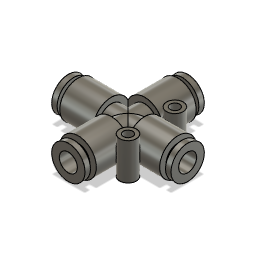
Top+Hydraulics (Autodesk Fusion 360 archive; units mm, degrees)
design "Cross Tube Fitting"
Autodesk Fusion 360 part; units mm, degrees
sketch "Sketch1" plane through (0, 0, 0) normal (0, 1, 0) x (1, 0, 0)
  line L0 (0, 21) -> (0, 0)
  line L1 (0, 21) -> (-5.875, 21)
  line L2 (-5.875, 21) -> (-5.875, 19.08)
  line L3 (-5.875, 19.08) -> (-4.175, 19.08)
  line L4 (-4.175, 19.08) -> (-4.175, 17.58)
  line L5 (-4.175, 17.58) -> (-6.45, 17.58)
  line L6 (-6.45, 17.58) -> (-6.45, 5.88)
  line L7 (-6.45, 5.88) -> (-4.475, 5.88)
  line L8 (-4.475, 5.88) -> (-4.475, 0)
  line L9 (-4.475, 0) -> (0, 0)
  line L10 (2.5, 0) -> (20, 0)
  line L11 (-5.875, -21) -> (-5.875, -19.08)
  line L12 (-6.45, -17.58) -> (-6.45, -5.88)
  line L13 (-4.175, -19.08) -> (-4.175, -17.58)
  line L14 (-5.875, -19.08) -> (-4.175, -19.08)
  line L15 (-6.45, -5.88) -> (-4.475, -5.88)
  line L16 (0, -21) -> (-5.875, -21)
  line L17 (-4.175, -17.58) -> (-6.45, -17.58)
  line L18 (0, -21) -> (0, 0)
  line L19 (-4.475, -5.88) -> (-4.475, 0)
  dimension "d1" = 21
  dimension "d2" = 5.875
  dimension "d3" = 1.92
  dimension "d4" = 1.7
  dimension "d5" = 1.5
  dimension "d6" = 2.275
  dimension "d7" = 11.7
  dimension "d8" = 5.88
  dimension "d9" = 4.475
  constraint coincident L0.end L9.end
  constraint perpendicular L0 L1
  constraint perpendicular L1 L2
  constraint perpendicular L2 L3
  constraint perpendicular L3 L4
  constraint perpendicular L4 L5
  constraint perpendicular L5 L6
  constraint perpendicular L6 L7
  constraint perpendicular L0 L9
  constraint parallel L9 L10
  constraint symmetric L0.start L9 L16.start
  constraint symmetric L0.end L9 L18.end
  constraint symmetric L1.end L9 L11.start
  constraint symmetric L2.end L9 L11.end
  constraint symmetric L3.end L9 L13.start
  constraint symmetric L4.end L9 L13.end
  constraint symmetric L5.end L9 L12.start
  constraint symmetric L6.end L9 L12.end
  constraint symmetric L7.end L9 L15.end
  constraint symmetric L8.end L9 L19.end
  measures "d1" distance of L0.start L0.end
  measures "d2" distance of L0.start L1.end
  measures "d3" distance of L1.end L2.end
  measures "d4" distance of L2.end L3.end
  measures "d5" distance of L3.end L4.end
  measures "d6" distance of L4.end L5.end
  measures "d7" distance of L5.end L6.end
  measures "d8" distance of L7.end L8.end
  measures "d9" distance of L0.end L8.end
revolve "Revolve1" add sketch "Sketch1" angle 360 about axis through (0, 0, 21) along (0, 0, -1)
sketch "Sketch2" plane through (0, 0, 0) normal (0, 1, 0) x (1, 0, 0)
  line L0 (19.08, 4.175) -> (17.58, 4.175)
  line L1 (5.88, 4.475) -> (0, 4.475)
  line L2 (21, 0) -> (21, 5.875)
  line L3 (21, 5.875) -> (19.08, 5.875)
  line L4 (5.88, 6.45) -> (5.88, 4.475)
  line L5 (0, 4.475) -> (0, 0)
  line L6 (17.58, 6.45) -> (5.88, 6.45)
  line L7 (21, 0) -> (0, 0)
  line L8 (17.58, 4.175) -> (17.58, 6.45)
  line L9 (19.08, 5.875) -> (19.08, 4.175)
  line L10 (0, 21) -> (0, 0)
  line L11 (-21, 0) -> (0, 0)
  line L12 (-17.58, 4.175) -> (-17.58, 6.45)
  line L13 (-5.88, 6.45) -> (-5.88, 4.475)
  line L14 (-19.08, 5.875) -> (-19.08, 4.175)
  line L15 (-17.58, 6.45) -> (-5.88, 6.45)
  line L16 (0, 4.475) -> (0, 0)
  line L17 (-19.08, 4.175) -> (-17.58, 4.175)
  line L18 (-21, 0) -> (-21, 5.875)
  line L19 (-21, 5.875) -> (-19.08, 5.875)
  line L20 (-5.88, 4.475) -> (0, 4.475)
  line L21 (2.5, 0) -> (20, 0)
  line L22 (0, -20) -> (0, -2.5)
  point P0 (0, 4.475)
  point P1 (0, 4.475)
  dimension "d11" = 21
  dimension "d12" = 5.875
  dimension "d13" = 1.92
  dimension "d14" = 1.7
  dimension "d15" = 1.5
  dimension "d16" = 2.275
  dimension "d17" = 11.7
  dimension "d18" = 5.88
  dimension "d19" = 4.475
  constraint coincident L5.end L7.end
  constraint perpendicular L2 L7
  constraint perpendicular L2 L3
  constraint perpendicular L3 L9
  constraint perpendicular L0 L9
  constraint perpendicular L0 L8
  constraint perpendicular L6 L8
  constraint perpendicular L4 L6
  constraint perpendicular L5 L7
  constraint symmetric L7.end L10.end L5
  constraint symmetric P1 P0 L5
  constraint symmetric L5.end L10 L7.end
  constraint symmetric L1.start L10 L13.end
  constraint symmetric L4.start L10 L13.start
  constraint symmetric L0.end L10 L12.start
  constraint symmetric L2.start L10 L11.start
  constraint symmetric L0.start L10 L14.end
  constraint symmetric L2.end L10 L18.end
  constraint symmetric L3.end L10 L14.start
  constraint symmetric P1 L10 P0
  constraint symmetric L6.start L10 L12.end
  constraint parallel L7 L11
  measures "d11" distance of L2.start L5.end
  measures "d12" distance of L2.start L2.end
  measures "d13" distance of L2.end L3.end
  measures "d14" distance of L0.start L3.end
  measures "d15" distance of L0.end L0.start
  measures "d16" distance of L0.end L6.start
  measures "d17" distance of L4.start L6.start
  measures "d18" distance of L1.start P0
  measures "d19" distance of P1 L5.end
revolve "Revolve2" add sketch "Sketch2" angle 360 about axis through (21, 0, 0) along (-1, 0, 0)
sketch "Sketch3" plane through (21, 0, 0) normal (1, 0, 0) x (0, 0, -1)
  circle A0 centre (0, 0) radius 5.875
  circle A1 centre (0, 0) radius 3.175
  dimension "d21" = 6.35
  constraint coincident A0.centre A1.centre
  measures "d21" diameter of A1
extrude "Extrude1" cut sketch "Sketch3" against normal up to surface (42 mm away) contours A1
sketch "Sketch4" plane through (0, 0, -21) normal (0, 0, -1) x (-1, 0, 0)
  circle A0 centre (0, 0) radius 5.875
  circle A1 centre (0, 0) radius 3.175
  dimension "d24" = 6.35
  constraint coincident A0.centre A1.centre
  measures "d24" diameter of A1
extrude "Extrude2" cut sketch "Sketch4" against normal up to surface (42 mm away) contours A1
sketch "Sketch5" plane through (0, 0, 0) normal (0, 1, 0) x (1, 0, 0)
  line L0 (0, -20) -> (0, -2.5)
  circle A0 centre (8.25, -8.25) radius 1.65
  line L1 (2.5, 0) -> (20, 0)
  circle A1 centre (8.25, -8.25) radius 2.95
  circle A2 centre (8.25, 8.25) radius 1.65
  circle A3 centre (8.25, 8.25) radius 2.95
  dimension "d27" = 3.3
  dimension "d28" = 8.25
  dimension "d29" = 8.25
  dimension "d30" = 5.9
  constraint concentric A0 A1
  constraint symmetric A0 L1 A2
  constraint symmetric L1 A1 A3
  measures "d27" diameter of A0
  measures "d28" distance of L0 A0.centre
  measures "d29" distance of A0.centre L1
  measures "d30" diameter of A1
extrude "Extrude3" add sketch "Sketch5" along normal mid plane 12.9

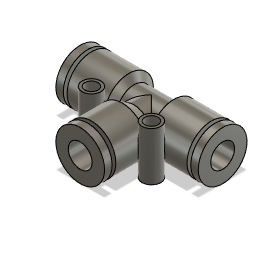
design "Marine 3-Way Push-to-Connect"
Autodesk Fusion 360 part; units mm, degrees
sketch "Sketch1" plane through (0, 0, 0) normal (0, 1, 0) x (1, 0, 0)
  line L0 (0, -20) -> (0, -2.5)
  line L1 (0, 3.18) -> (19, 3.18)
  line L2 (2.5, 0) -> (20, 0)
  line L3 (19, 3.18) -> (19, 6.5)
  line L4 (0, 4.55) -> (4.65, 4.55)
  line L5 (4.65, 4.55) -> (6, 6.5)
  line L6 (17, 6.5) -> (17, 3.75)
  line L7 (17, 3.75) -> (16, 3.75)
  line L8 (16, 3.75) -> (16, 6.5)
  line L9 (19, 6.5) -> (17, 6.5)
  line L10 (16, 6.5) -> (6, 6.5)
  line L11 (0, 4.55) -> (-4.65, 4.55)
  line L12 (0, 3.18) -> (-19, 3.18)
  line L13 (-4.65, 4.55) -> (-6, 6.5)
  line L14 (-16, 6.5) -> (-6, 6.5)
  line L15 (-16, 3.75) -> (-16, 6.5)
  line L16 (-17, 6.5) -> (-17, 3.75)
  line L17 (-17, 3.75) -> (-16, 3.75)
  line L18 (-19, 6.5) -> (-17, 6.5)
  line L19 (-19, 3.18) -> (-19, 6.5)
  dimension "d2" = 19
  dimension "d3" = 3.18
  dimension "d4" = 6.5
  dimension "d5" = 6
  dimension "d6" = 4.65
  dimension "d7" = 4.55
  dimension "d8" = 1
  dimension "d9" = 2
  dimension "d10" = 2.75
  constraint horizontal L1
  constraint coincident L0 L1.start
  constraint perpendicular L1 L3
  constraint perpendicular L3 L9
  constraint horizontal L4
  constraint perpendicular L6 L9
  constraint perpendicular L3 L7
  constraint coincident L8.end L9
  constraint perpendicular L8 L9
  constraint collinear L9 L10
  constraint symmetric L0 L1.start L12.start
  constraint symmetric L0 L1.end L12.end
  constraint symmetric L0 L3.end L18.start
  constraint symmetric L0 L5.end L13.end
  constraint symmetric L0 L4.start L11.start
  constraint symmetric L0 L4.end L11.end
  constraint symmetric L0 L6.start L16.start
  constraint symmetric L0 L6.end L16.end
  constraint symmetric L0 L7.end L15.start
  constraint symmetric L0 L8.end L14.start
  constraint coincident L4.start L11.start
  measures "d2" distance of L1.start L1.end
  measures "d3" distance of L1 L2
  measures "d4" distance of L2 L3.end
  measures "d5" distance of L0 L5.end
  measures "d6" distance of L4.start L4.end
  measures "d7" distance of L2 L4
  measures "d8" distance of L6.end L7.end
  measures "d9" distance of L3.end L6.start
  measures "d10" distance of L6.start L6.end
revolve "Revolve1" add sketch "Sketch1" angle 360 about axis through (2.5, 0, 0) along (1, 0, 0)
sketch "Sketch2" plane through (0, 0, 0) normal (0, 1, 0) x (1, 0, 0)
  line L0 (3.75, -16) -> (6.5, -16)
  line L1 (3.18, -19) -> (6.5, -19)
  line L2 (4.55, -4.65) -> (6.5, -7.75)
  line L3 (4.55, 0) -> (4.55, -4.65)
  line L4 (3.18, 0) -> (3.18, -19)
  line L5 (6.5, -17) -> (3.75, -17)
  line L6 (6.5, -19) -> (6.5, -17)
  line L7 (6.5, -16) -> (6.5, -7.75)
  line L8 (3.75, -17) -> (3.75, -16)
  line L9 (0, -20) -> (0, -2.5)
  line L10 (4.55, 0) -> (3.18, 0)
  line L11 (2.5, 0) -> (20, 0)
  dimension "d12" = 19
  dimension "d13" = 4.65
  dimension "d14" = 1
  dimension "d15" = 2
  dimension "d16" = 2.75
  dimension "d17" = 3.18
  dimension "d18" = 6.5
  dimension "d19" = 4.55
  dimension "d20" = 8.25
  constraint perpendicular L1 L4
  constraint perpendicular L1 L6
  constraint perpendicular L5 L6
  constraint perpendicular L1 L8
  constraint coincident L0.end L6
  constraint perpendicular L0 L6
  constraint collinear L6 L7
  constraint parallel L4 L9
  constraint perpendicular L3 L10
  constraint coincident L4.start L11
  measures "d12" distance of L1.start L4.start
  measures "d13" distance of L3.start L2.start
  measures "d14" distance of L0.start L5.end
  measures "d15" distance of L5.start L1.end
  measures "d16" distance of L5.start L5.end
  measures "d17" distance of L4 L9
  measures "d18" distance of L7 L9
  measures "d19" distance of L3 L9
  measures "d20" distance of L2.end L0.end
revolve "Revolve2" add sketch "Sketch2" angle 360 about axis through (0, 0, 20) along (0, 0, -1)
sketch "Sketch3" plane through (19, 0, 0) normal (1, 0, 0) x (0, 0, -1)
  circle A0 centre (0, 0) radius 6.5
  circle A1 centre (0, 0) radius 3.18
  circle A2 centre (0, 0) radius 3.18
extrude "Extrude1" cut sketch "Sketch3" against normal up to surface (38 mm away) contours A1 A2
sketch "Sketch4" plane through (0, 0, 19) normal (0, 0, 1) x (1, 0, 0)
  circle A0 centre (0, 0) radius 6.5
  circle A1 centre (0, 0) radius 3.18
  circle A2 centre (0, 0) radius 3.18
extrude "Extrude2" cut sketch "Sketch4" along normal up to surface contours A1 A2 end surface at (-12.6667, 3.1455, -0.4668)
ref_plane "WorkPlane1" through (0, 6.5, 0) normal (0, 1, 0) x (0, 0, 1)
sketch "Sketch5" plane through (0, 6.5, 0) normal (0, 1, 0) x (1, 0, 0)
  line L0 (0, -20) -> (0, -2.5)
  line L1 (2.5, 0) -> (20, 0)
  circle A0 centre (8, -8) radius 1.75
  circle A1 centre (8, -8) radius 2.5
  circle A2 centre (-8, -8) radius 2.5
  circle A3 centre (-8, -8) radius 1.75
  dimension "d27" = 8
  dimension "d28" = 8
  dimension "d29" = 3.5
  dimension "d30" = 5
  constraint concentric A0 A1
  constraint symmetric L0 A0 A3
  constraint symmetric L0 A1 A2
  measures "d27" distance of L1 A0.centre
  measures "d28" distance of L0 A0.centre
  measures "d29" diameter of A0
  measures "d30" diameter of A1
extrude "Extrude3" add sketch "Sketch5" against normal blind 13
extrude "Extrude4" cut sketch "Sketch5" against normal up to surface (13 mm away) contours A0 | A3
